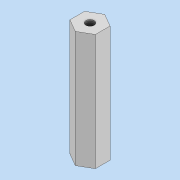
# Autodesk Inventor part: HexShaft
Saved by Autodesk Inventor 2022 (Build 260153000, 153)
## iProperties
Created: 2023-02-11
Part Number: HexShaft
Material: Generic
Document SubType Name: Modeling
Designer: coled
Density: 1 g/cm^3
Appearance: Default
Author: coled
Autodesk Inventor part; units mm, degrees
ref_plane "YZ Plane" through (0, 0, 0) normal (1, 0, 0) x (0, 1, 0)
ref_plane "XZ Plane" through (0, 0, 0) normal (0, 1, 0) x (-1, 0, 0)
ref_plane "XY Plane" through (0, 0, 0) normal (0, 0, 1) x (1, 0, 0)
sketch "Sketch1" plane through (0, 0, 0) normal (0, 1, 0) x (-1, 0, 0)
  line L0 (0, 0) -> (6.35, 0)
  line L1 (6.35, -3.6662) -> (0, -7.3323)
  line L2 (0, -7.3323) -> (-6.35, -3.6662)
  line L3 (-6.35, -3.6662) -> (-6.35, 3.6662)
  line L4 (-6.35, 3.6662) -> (0, 7.3323)
  line L5 (0, 7.3323) -> (6.35, 3.6662)
  line L6 (6.35, 3.6662) -> (6.35, -3.6662)
  dimension "d0" = 6.35
  constraints: 14 end point, 1 coincident, 1 horizontal, 1 midpoint, 13 other
  measures "d0" distance of L0.start L0.end
extrude "Extrusion1" add sketch "Sketch1" along normal blind 58
sketch "Sketch3" plane through (0, 58, 0) normal (0, 1, 0) x (1, 0, 0)
  point P0 (0, 0)
  point P1 (0, 0)
  constraints: 1 coincident
hole "Hole1" at (0, 58, 0) direction (0, -1, 0) diameter 4.134 depth 13 tip angle 118 thread size "M5x0.8" class "6H" standard "ANSI Metric M Profile"
sketch "Sketch4" plane through (0, 0, 0) normal (0, -1, 0) x (1, 0, 0)
  point P0 (0, 0)
  point P1 (0, 0)
  constraints: 1 coincident
hole "Hole2" at (0, 0, 0) direction (0, 1, 0) diameter 4.134 depth 13 tip angle 118 thread size "M5x0.8" class "6H" standard "ANSI Metric M Profile"
body "Solid1"
